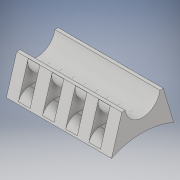
# Autodesk Inventor part: Sensor_platform
Saved by Autodesk Inventor 2017 (Build 210142000, 142)
## iProperties
Created: 2018-06-16
Part Number: Sensor_platform
Material: Generic
Document SubType Name: Modeling
Designer: Arthur
Density: 1 g/cm^3
Appearance: Default
Author: Arthur
Autodesk Inventor part; units mm, degrees
ref_plane "YZ Plane" through (0, 0, 0) normal (1, 0, 0) x (0, 1, 0)
ref_plane "XZ Plane" through (0, 0, 0) normal (0, 1, 0) x (-1, 0, 0)
ref_plane "XY Plane" through (0, 0, 0) normal (0, 0, 1) x (1, 0, 0)
sketch "Sketch1" plane through (0, 0, 0) normal (1, 0, 0) x (0, 1, 0)
  line L0 (10.5, 18.75) -> (-10.5, 18.75)
  line L1 (-10.5, 18.75) -> (-10.5, -18.75)
  line L2 (-10.5, -18.75) -> (10.5, -18.75)
  line L3 (10.5, -18.75) -> (10.5, 18.75)
  constraints: 8 end point, 2 parallel, 1 horizontal, 1 perpendicular
extrude "Extrusion1" add sketch "Sketch1" along normal blind 63.5
sketch "Sketch2" plane through (63.5, 0, 0) normal (1, 0, 0) x (0, 0, -1)
  line L0 (-18.75, -10.5) -> (18.75, -10.5) projected
  line L1 (18.75, -10.5) -> (-18.75, -10.5)
  line L2 (-18.75, 10.5) -> (-18.75, -10.5) projected
  arc A0 (18.75, -10.5) -> (-18.75, -10.5) centre (0, -50.857) ccw
  point P0 (0, 0)
  dimension "d4" = 44.5
  constraints: 2 end point, 2 point on circle, 1 centre point, 1 collinear
  measures "d4" radius of A0
extrude "Extrusion2" cut sketch "Sketch2" against normal through all
sketch "Sketch3" plane through (63.5, 0, 0) normal (1, 0, 0) x (0, 0, -1)
  line L0 (0, 10.5) -> (10.5, 10.5)
  line L1 (0, 10.5) -> (-10.5, 10.5)
  arc A0 (-10.5, 10.5) -> (10.5, 10.5) centre (0, 12.125) ccw
  line L2 (12.5, 10.5) -> (18.75, -10.5)
  line L3 (18.75, -10.5) -> (18.75, 10.5) projected
  line L4 (18.75, -10.5) -> (18.75, 10.5)
  line L5 (18.75, 10.5) -> (12.5, 10.5)
  line L6 (18.75, 10.5) -> (-18.75, 10.5) projected
  line L7 (-18.75, 10.5) -> (-18.75, -10.5) projected
  line L8 (-12.5, 10.5) -> (-18.75, -10.5)
  line L9 (-18.75, -10.5) -> (-18.75, 10.5)
  line L10 (-18.75, 10.5) -> (-12.5, 10.5)
  dimension "d11" = 10.5
  dimension "d12" = 10.5
  dimension "d14" = 2
  dimension "d15" = 2
  constraints: 16 end point, 2 perpendicular, 2 point on circle, 1 centre point, 1 collinear, 1 point on line
  measures "d11" distance of L0.start L0.end
  measures "d12" distance of L0.start L1.end
  measures "d14" distance of L0.end L2.start
  measures "d15" distance of L1.end L8.start
extrude "Extrusion3" cut sketch "Sketch3" against normal through all
sketch "Sketch4" plane through (0, -10.5, 18.75) normal (0, 0.2852536, 0.9584521) x (1, 0, 0)
  line L0 (56.5, 6.4322) -> (49.5, 6.4322)
  line L1 (49.5, 6.4322) -> (49.5, 12.4322)
  line L2 (49.5, 12.4322) -> (56.5, 12.4322)
  line L3 (56.5, 12.4322) -> (56.5, 6.4322)
  line L4 (42.5, 6.4322) -> (35.5, 6.4322)
  line L5 (35.5, 6.4322) -> (35.5, 12.4322)
  line L6 (35.5, 12.4322) -> (42.5, 12.4322)
  line L7 (42.5, 12.4322) -> (42.5, 6.4322)
  line L8 (28.5, 6.4322) -> (21.5, 6.4322)
  line L9 (21.5, 6.4322) -> (21.5, 12.4322)
  line L10 (21.5, 12.4322) -> (28.5, 12.4322)
  line L11 (28.5, 12.4322) -> (28.5, 6.4322)
  line L12 (13.9988, 6.4322) -> (6.9988, 6.4322)
  line L13 (6.9988, 6.4322) -> (6.9988, 12.4322)
  line L14 (6.9988, 12.4322) -> (13.9988, 12.4322)
  line L15 (13.9988, 12.4322) -> (13.9988, 6.4322)
  point P0 (0, 15.4123)
  dimension "d20" = 7
  dimension "d21" = 6
  dimension "d23" = 7
  dimension "d24" = 6
  dimension "d27" = 7
  dimension "d28" = 6
  dimension "d29" = 7
  dimension "d30" = 6
  constraints: 32 end point, 8 parallel, 4 horizontal, 4 perpendicular
  measures "d20" distance of L1.end L2.end
  measures "d21" distance of L0.end L1.end
  measures "d23" distance of L6.start L6.end
  measures "d24" distance of L4.end L6.start
  measures "d27" distance of L10.start L10.end
  measures "d28" distance of L8.end L10.start
  measures "d29" distance of L14.start L14.end
  measures "d30" distance of L12.end L14.start
sketch "Sketch6" plane through (0, 10.5, 12.5) normal (0, 1, 0) x (1, 0, 0)
  line L0 (52.4994, -12.5655) -> (52.4994, 39.8038)
  line L1 (39.4491, -12.5655) -> (39.4491, 40.8679)
  line L2 (24.9507, -12.5655) -> (24.9507, 40.8679)
  line L3 (10.5396, -12.5655) -> (10.5396, 40.8679)
  point P0 (0, 12.5)
  constraints: 8 end point, 4 vertical
sweep "Sweep1" cut profiles "Sketch4" path "Sketch6" path curves L1
fillet "Fillet1" radius 7 8 edges at (39, 1.4157, 15.2037) (53, 1.4157, 15.2037) (25, 1.4157, 15.2037) (10.4988, 1.4157, 15.2037) (53, 1.4157, -15.2037) (39, 1.4157, -15.2037) (25, 1.4157, -15.2037) (10.4988, 1.4157, -15.2037)
fillet "Fillet2" radius 7 8 edges at (53, -4.335, 16.9152) (39, -4.335, 16.9152) (25, -4.335, 16.9152) (10.4988, -4.335, 16.9152) (53, -4.335, -16.9152) (39, -4.335, -16.9152) (25, -4.335, -16.9152) (10.4988, -4.335, -16.9152)
body "Solid1"
